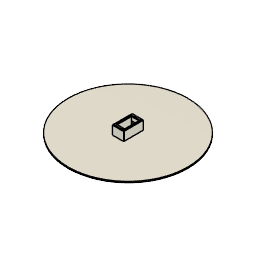
Davinki Assembly (Autodesk Fusion 360 archive; units mm, degrees)
design "Davinki Base"
part number: 2026-08-29-10-07-06-773
Autodesk Fusion 360 part; units mm, degrees
sketch "Sketch1" plane through (0, 0, 0) normal (0, 1, 0) x (1, 0, 0)
  line L0 (0, 0) -> (12.25, 0)
  line L1 (12.25, 0) -> (12.25, 23.5)
  line L2 (0, 0) -> (0, 23.5)
  line L3 (0, 23.5) -> (12.25, 23.5)
  line L4 (-3.4056, 0) -> (-3.4056, 27)
  line L5 (-3.4056, 27) -> (15.0988, 27)
  line L6 (15.0988, 27) -> (15.0988, -3.5)
  line L7 (15.0988, -3.5) -> (-3.4056, -3.5)
  line L8 (-3.4056, -3.5) -> (-3.4056, 27)
  line L9 (-3.4056, 27) -> (-3.4056, 28)
  line L10 (-3.4056, 28) -> (15.0988, 28)
  line L11 (15.0988, 28) -> (15.0988, 27)
  line L12 (-3.4056, -3.5) -> (-3.4056, -4.5)
  line L13 (-3.4056, -4.5) -> (15.1, -4.5)
  line L14 (15.1, -4.5) -> (15.0988, -3.5)
  line L15 (0, 23.5) -> (0, 0.25)
  line L16 (12.25, 11.75) -> (-3.4056, 11.75)
  line L17 (0.8466, 88) -> (10.8466, 88)
  line L18 (10.8472, -64.5) -> (0.8466, -64.5)
  circle A0 centre (5.9954, 11.75) radius 18.8312
  circle A1 centre (5.9954, 11.75) radius 98.6653
  dimension "d1" = 12.25
  dimension "d2" = 23.5
  dimension "d3" = 23.5
  dimension "d6" = 30.5
  dimension "d7" = 1
  dimension "d8" = 1
  dimension "d16" = 23.25
  constraint coincident L0.start L2.start
  constraint horizontal L0
  constraint perpendicular L0 L1
  constraint perpendicular L0 L2
  constraint horizontal L5
  constraint vertical L6
  constraint horizontal L7
  constraint vertical L8
  constraint perpendicular L5 L9
  constraint perpendicular L6 L10
  constraint perpendicular L5 L11
  constraint perpendicular L7 L12
  constraint perpendicular L8 L13
  constraint perpendicular L0 L15
  constraint midpoint L1 L16.start
  constraint midpoint L8 L16.end
  constraint perpendicular L4 L16
  constraint coincident L16 A0.centre
  constraint concentric A0 A1
  measures "d1" distance of L0.start L0.end
  measures "d2" distance of L0.end L1.end
  measures "d3" distance of L0.start L2.end
  measures "d6" distance of L4.end L7.end
  measures "d7" distance of L4.end L9.end
  measures "d8" distance of L7.end L12.end
  measures "d16" distance of L2.end L15.end
extrude "Extrude1" add sketch "Sketch1" along normal blind 17.3 contours L4 L5 L6 L7 L8 | L7 L12 L13 L14 | L5 L9 L10 L11
sketch "Sketch2" plane through (0, 0, -28) normal (0, 0, -1) x (-1, 0, 0)
  line L0 (-15.0988, 0) -> (3.4056, 0)
  line L1 (3.4056, 0) -> (3.4056, 17.3)
  line L2 (3.4056, 17.3) -> (-15.0988, 17.3)
  line L3 (-15.0988, 17.3) -> (-15.0988, 0)
  line L4 (-11.5, 2) -> (-1.0253, 2)
  line L5 (-1.0253, 2) -> (-1.0253, 5)
  line L6 (-11.5, 5) -> (-11.5, 2)
  line L7 (-11.5, 5) -> (-11.5, 10)
  line L8 (-11.5, 10) -> (-1, 10)
  line L9 (-1, 10) -> (-1.0253, 5)
  dimension "d11" = 3
  constraint horizontal L4
  constraint vertical L5
  constraint vertical L6
  constraint perpendicular L7 L8
  measures "d11" distance of L4.start L6.start
extrude "Extrude2" cut sketch "Sketch2" against normal blind 16 contours L4 L5 L6 L7 L8 L9
fillet "Fillet1" radius 1 1 faces at (3.8981, 17.3, 3)
extrude "Extrude6" add sketch "Sketch1" along normal blind 2 contours A0 | A1
